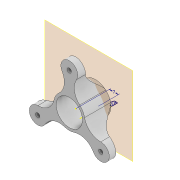
# Autodesk Inventor part: elektromagneet
Saved by Autodesk Inventor 2020.3 (Build 243373000, 373)
## iProperties
Created: 2020-06-22
Part Number: elektromagneet
Material: Generic
Document SubType Name: Modeling
Designer: Svend
Density: 1 g/cm^3
Appearance: Default
Author: Svend
Autodesk Inventor part; units mm, degrees
ref_plane "YZ Plane" through (0, 0, 0) normal (1, 0, 0) x (0, 1, 0)
ref_plane "XZ Plane" through (0, 0, 0) normal (0, 1, 0) x (-1, 0, 0)
ref_plane "XY Plane" through (0, 0, 0) normal (0, 0, 1) x (1, 0, 0)
ref_plane "Work Plane1" through (0, 0, 0) normal (0, 0, 1) x (1, 0, 0)
sketch "Sketch1" plane through (0, 0, 0) normal (0, 0, 1) x (1, 0, 0)
  circle A0 centre (0, -28) radius 1.621 projected
  circle A1 centre (-24.2487, -14) radius 1.621 projected
  circle A2 centre (-24.2487, 14) radius 1.621 projected
  circle A3 centre (0, 28) radius 1.621 projected
  circle A4 centre (24.2487, 14) radius 1.621 projected
  circle A5 centre (24.2487, -14) radius 1.621 projected
  circle A6 centre (28, 0) radius 1.621 projected
  circle A7 centre (14, 24.2487) radius 1.621 projected
  circle A8 centre (-14, 24.2487) radius 1.621 projected
  circle A9 centre (-28, 0) radius 1.621 projected
  circle A10 centre (-14, -24.2487) radius 1.621 projected
  circle A11 centre (14, -24.2487) radius 1.621 projected
  circle A12 centre (6, -10.3923) radius 4.55 projected
  circle A13 centre (0, 0) radius 4.5 projected
  circle A14 centre (0, 0) radius 34.5 projected
  circle A15 centre (6, 10.3923) radius 4.55 projected
  circle A16 centre (-12, 0) radius 4.55 projected
  circle A17 centre (0, 0) radius 35 projected
  point P0 (0, 0)
extrude "Extrusion1" add sketch "Sketch1" along normal blind 5 contours A0 | A2 | A4 | A6 | A7 | A8 | A9 | A10 | A11 | A12 | A13 | A14 | A15 | A16
sketch "Sketch2" plane through (0, 0, 0) normal (0, 0, -1) x (-1, 0, 0)
  circle A0 centre (0, 0) radius 34.5 projected
  circle A1 centre (-24.2487, -14) radius 1.621 projected
  circle A2 centre (0, 28) radius 1.621 projected
  circle A3 centre (24.2487, -14) radius 1.621 projected
  circle A4 centre (0, 0) radius 10.1
  circle A5 centre (0, 0) radius 12
  point P0 (0, 0)
  dimension "d2" = 20.2
  dimension "d3" = 24
  constraints: 2 centre point, 2 coincident
  measures "d2" diameter of A4
  measures "d3" diameter of A5
extrude "Extrusion2" add sketch "Sketch2" along normal blind 15 contours A5
sketch "Sketch3" plane through (0, 0, 0) normal (1, 0, 0) x (0, 1, 0)
  line L0 (12, 0) -> (12, -15) projected
  line L1 (-12, -15) -> (12, -15) projected
  line L2 (12, 0) -> (-12, 0) projected
  line L3 (34.5, 5) -> (-34.5, 5) projected
  line L4 (34.5, 0) -> (-34.5, 0) projected
  line L5 (34.5, 0) -> (-34.5, 0) projected
  arc A0 (34.5, 0) -> (12, -15) centre (34.5, -24.375) ccw
  line L6 (0, -30.25) -> (0, 10.875) projected
  point P0 (0, 0)
  point P1 (12, -15)
  constraints: 2 point on circle, 1 centre point, 1 tangent
revolve "Revolution1" add sketch "Sketch3" angle 360 about axis through (0, 0, -10) along (0, 0, 1) contours L4 A0 L0
sketch "Sketch4" plane through (0, 0, 5) normal (0, 0, 1) x (1, 0, 0)
  circle A0 centre (0, 0) radius 34.5 projected
  circle A1 centre (24.2487, -14) radius 1.621 projected
  circle A2 centre (0, 28) radius 1.621 projected
  circle A3 centre (-24.2487, -14) radius 1.621 projected
  point P0 (0, 0)
extrude "Extrusion3" cut sketch "Sketch4" against normal through all contours A1 | A2 | A3
sketch "Sketch5" plane through (0, 0, 5) normal (0, 0, 1) x (1, 0, 0)
  circle A0 centre (0, 0) radius 12 projected
  circle A1 centre (-24.2487, -14) radius 1.621 projected
  circle A2 centre (24.2487, -14) radius 1.621 projected
  circle A3 centre (0, 28) radius 1.621 projected
  circle A4 centre (-24.2487, -14) radius 6.5
  circle A5 centre (0, 28) radius 6.5
  circle A6 centre (24.2487, -14) radius 6.5
  circle A7 centre (0, 0) radius 34.5 projected
  arc A8 (18.5749, -17.1715) -> (3.7537, -11.3978) centre (7.6638, -23.2705) ccw
  arc A9 (11.7476, 2.4481) -> (24.1584, -7.5006) centre (23.9848, 4.9982) ccw
  arc A10 (5.5835, 24.6721) -> (7.9939, 8.9497) centre (16.3209, 18.2723) ccw
  arc A11 (-7.9939, 8.9497) -> (-5.5835, 24.6721) centre (-16.3209, 18.2723) ccw
  arc A12 (-24.1584, -7.5006) -> (-11.7476, 2.4481) centre (-23.9848, 4.9982) ccw
  arc A13 (-3.7537, -11.3978) -> (-18.5749, -17.1715) centre (-7.6638, -23.2705) ccw
  point P0 (0, 0)
  point P1 (-3.7537, -11.3978)
  point P2 (-18.5749, -17.1715)
  point P3 (-29.8779, -17.25)
  point P4 (29.8779, -17.25)
  point P5 (-11.7476, 2.4481)
  point P6 (-7.9939, 8.9497)
  point P7 (-5.5835, 24.6721)
  point P8 (0, 34.5)
  point P9 (5.5835, 24.6721)
  point P10 (7.9939, 8.9497)
  dimension "d9" = 12.5
  dimension "d12" = 360
  constraints: 16 point on circle, 9 centre point, 7 tangent, 3 coincident, 1 equal radius, 25 other
  measures "d9" radius of A8
extrude "Extrusion4" cut sketch "Sketch5" against normal through all contours A0 A10 A5 A7 A6 A9 | A8 A6 A7 A4 A13 A0 | A0 A12 A4 A7 A5 A11
sketch "Sketch6" plane through (0, 0, 0) normal (0, 0, -1) x (-1, 0, 0)
  circle A0 centre (0, 0) radius 10.1 projected
  point P0 (0, 0)
extrude "Extrusion5" cut sketch "Sketch6" against normal through all
ref_plane "Work Plane2" through (0, 0, -10) normal (0, 0, 1) x (1, 0, 0)
sketch "Sketch7" plane through (0, 0, -10) normal (0, 0, 1) x (1, 0, 0)
  circle A0 centre (0, 0) radius 10.1 projected
  circle A1 centre (0, 0) radius 10.1 projected
  circle A2 centre (0, 0) radius 10.1 projected
  circle A3 centre (0, 0) radius 8.25
  point P0 (0, 0)
  dimension "d19" = 16.5
  constraints: 1 centre point, 1 coincident
  measures "d19" diameter of A3
extrude "Extrusion6" add sketch "Sketch7" against normal up to surface (5 mm away)
sketch "Sketch8" plane through (0, 0, 0) normal (0, 1, 0) x (-1, 0, 0)
  line L0 (-8.25, -15) -> (-8.25, -10) projected
  line L1 (-10.1, -10) -> (10.1, -10) projected
  line L2 (-11.7476, -15) -> (-7.9939, -15) projected
  line L3 (-8.25, -15) -> (-7, -10)
  line L4 (-7, -10) -> (-8.25, -10)
  line L5 (-7.9939, 5) -> (-7.9939, -15) projected
  line L6 (-8.25, -15) -> (-9.5, -20)
  line L7 (-9.5, -20) -> (-12, -20)
  line L8 (-12, -15) -> (-3.7537, -15) projected
  line L9 (-12, -20) -> (-12, -15)
  point P0 (0, 0)
  dimension "d22" = 7
  dimension "d23" = 5
  constraints: 10 end point, 1 collinear, 1 horizontal, 1 parallel, 1 perpendicular, 1 point on line
  measures "d22" horizontal distance of point (0, 0) L3.end
  measures "d23" distance between parallel lines of L2 L7
body "Solid1"
